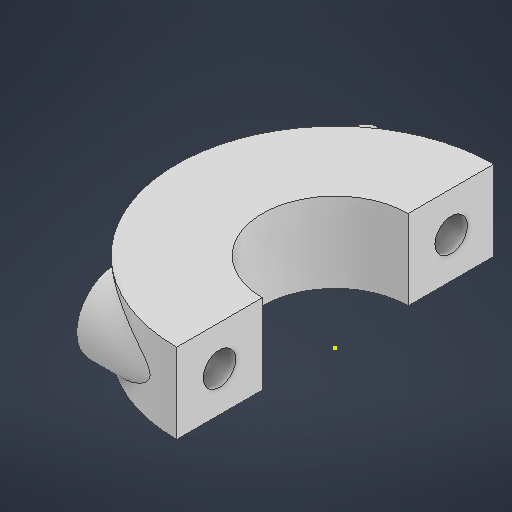
# Autodesk Inventor part: clamp_bolt
Saved by Autodesk Inventor 2026.2 (Build 302298000, 298)
## iProperties
Created: 2026-01-11
Part Number: clamp_bolt
Material: Generic
Document SubType Name: Modeling
Designer: User
Density: 1 g/cm^3
Appearance: Default
Author: User
Autodesk Inventor part; units mm, degrees
ref_plane "YZ Plane" through (0, 0, 0) normal (1, 0, 0) x (0, 1, 0)
ref_plane "XZ Plane" through (0, 0, 0) normal (0, 1, 0) x (-1, 0, 0)
ref_plane "XY Plane" through (0, 0, 0) normal (0, 0, 1) x (1, 0, 0)
sketch "Sketch1" plane through (0, 0, 0) normal (0, 1, 0) x (-1, 0, 0)
  point P0 (0, 0)
sketch "Sketch2" plane through (0, 0, 0) normal (0, 1, 0) x (-1, 0, 0)
  arc A0 (0, -12.775) -> (0, 12.775) centre (0, 0) ccw
  arc A1 (0, -27.775) -> (0, 27.775) centre (0, 0) ccw
  line L0 (0, 27.775) -> (0, -27.775)
  dimension "d0" = 25.55
  dimension "d1" = 15
  constraints: 4 point on circle, 2 centre point, 2 end point, 2 point on line, 1 coincident, 1 vertical
  measures "d0" diameter of A0
  measures "d1" radial gap between concentric circles of A0 A1
extrude "Extrusion1" add sketch "Sketch2" along normal blind 14 contours A0 L0 A1
sketch "Sketch4" plane through (0, 0, 27.775) normal (1, 0, 0) x (0, 0, -1)
  line L0 (4.7364, 11.7377) -> (10.2211, 11.7622)
  line L1 (10.2211, 11.7622) -> (12.9848, 7.0245)
  line L2 (12.9848, 7.0245) -> (10.2636, 2.2623)
  line L3 (10.2636, 2.2623) -> (4.7789, 2.2378)
  line L4 (4.7789, 2.2378) -> (2.0152, 6.9755)
  line L5 (2.0152, 6.9755) -> (4.7364, 11.7377)
  line L6 (0, 14) -> (15, 14) projected
  line L7 (0, 0) -> (0, 14) projected
  line L8 (15, 14) -> (40.55, 14) projected
  line L9 (27.775, 14) -> (27.775, 0)
  line L10 (50.8136, 11.7377) -> (45.3289, 11.7622)
  line L11 (45.3289, 11.7622) -> (42.5652, 7.0245)
  line L12 (42.5652, 7.0245) -> (45.2864, 2.2623)
  line L13 (45.2864, 2.2623) -> (50.7711, 2.2378)
  line L14 (50.7711, 2.2378) -> (53.5348, 6.9755)
  line L15 (53.5348, 6.9755) -> (50.8136, 11.7377)
  line L16 (55.55, 14) -> (40.55, 14)
  line L17 (55.55, 0) -> (55.55, 14)
  line L18 (40.55, 14) -> (15, 14)
  point P0 (7.5, 7)
  point P1 (7.4787, 11.75)
  point P2 (7.5, 14)
  point P3 (0, 7)
  point P4 (48.05, 7)
  point P5 (48.0713, 11.75)
  point P6 (48.05, 14)
  point P7 (55.55, 7)
  dimension "d5" = 9.5
  dimension "d6" = 0
  dimension "d7" = 0
  constraints: 32 end point, 14 symmetric about line, 4 midpoint, 1 vertical, 13 other
  measures "d5" distance from line of L3 point (7.479, 11.75)
  measures "d6" horizontal distance of point (7.5, 14) point (7.5, 7)
  measures "d7" vertical distance of point (0, 7) point (7.5, 7)
extrude "Extrusion2" cut sketch "Sketch4" against normal through all
sketch "Sketch5" plane through (0, 0, 27.775) normal (1, 0, 0) x (0, 0, -1)
  line L0 (4.7364, 11.7377) -> (10.2211, 11.7622) projected
  circle A0 centre (7.4787, 6.9999) radius 2.85
  line L1 (0.8522, 11.9261) -> (14.3606, 11.9261)
  line L2 (14.3606, 11.9261) -> (14.3606, 2.2036)
  line L3 (14.3606, 2.2036) -> (0.8522, 2.2036)
  line L4 (0.8522, 2.2036) -> (0.8522, 11.9261)
  line L5 (10.2636, 2.2623) -> (4.7789, 2.2378) projected
  line L6 (55.55, 14) -> (0, 14) projected
  line L7 (27.775, 14) -> (27.775, 0)
  line L8 (55.55, 0) -> (0, 0) projected
  line L9 (50.8136, 11.7377) -> (45.3289, 11.7622)
  circle A1 centre (48.0713, 6.9999) radius 2.85
  line L10 (54.6978, 11.9261) -> (41.1894, 11.9261)
  line L11 (41.1894, 11.9261) -> (41.1894, 2.2036)
  line L12 (41.1894, 2.2036) -> (54.6978, 2.2036)
  line L13 (54.6978, 2.2036) -> (54.6978, 11.9261)
  line L14 (45.2864, 2.2623) -> (50.7711, 2.2378)
  point P0 (7.4787, 11.75)
  point P1 (7.4787, 11.75)
  point P2 (48.0713, 11.75)
  point P3 (48.0713, 11.75)
  dimension "d12" = 5.7
  dimension "d13" = 0
  dimension "d14" = 4.75
  constraints: 22 end point, 11 symmetric about line, 4 midpoint, 2 centre point, 2 parallel, 1 horizontal, 1 perpendicular, 1 other
  measures "d12" diameter of A0
  measures "d13" horizontal distance of point (7.479, 11.75) A0.centre
  measures "d14" distance from line of L5 A0.centre
extrude "Extrusion3" add sketch "Sketch5" against normal blind 6
sketch "Sketch6" plane through (-6, 0, 27.775) normal (-1, 0, 0) x (0, 0, 1)
  line L0 (-27.775, 0) -> (-27.775, 14)
  line L1 (-40.55, 14) -> (-15, 14) projected
  line L2 (-10.2636, 2.2623) -> (-4.7789, 2.2378) projected
  line L3 (-10.2636, 2.2623) -> (-4.7789, 2.2378)
  line L4 (-4.7789, 2.2378) -> (-2.0152, 6.9755) projected
  line L5 (-4.7789, 2.2378) -> (-2.0152, 6.9755)
  line L6 (-2.0152, 6.9755) -> (-4.7364, 11.7377) projected
  line L7 (-2.0152, 6.9755) -> (-4.7364, 11.7377)
  line L8 (-4.7364, 11.7377) -> (-10.2636, 11.7624)
  line L9 (-10.2636, 11.7624) -> (-13.0059, 7.0615)
  line L10 (-13.0059, 7.0615) -> (-10.2636, 2.2623)
  circle A0 centre (-7.4787, 6.9999) radius 2.85 projected
  circle A1 centre (-7.4787, 6.9999) radius 7
  line L11 (-45.2864, 2.2623) -> (-50.7711, 2.2378)
  line L12 (-45.2864, 2.2623) -> (-50.7711, 2.2378)
  line L13 (-50.7711, 2.2378) -> (-53.5348, 6.9755)
  line L14 (-50.7711, 2.2378) -> (-53.5348, 6.9755)
  line L15 (-53.5348, 6.9755) -> (-50.8136, 11.7377)
  line L16 (-53.5348, 6.9755) -> (-50.8136, 11.7377)
  line L17 (-50.8136, 11.7377) -> (-45.2864, 11.7624)
  line L18 (-45.2864, 11.7624) -> (-42.5441, 7.0615)
  line L19 (-42.5441, 7.0615) -> (-45.2864, 2.2623)
  circle A2 centre (-48.0713, 6.9999) radius 2.85
  circle A3 centre (-48.0713, 6.9999) radius 7
  dimension "d17" = 14
  constraints: 32 end point, 8 symmetric about line, 3 centre point, 3 collinear, 3 parallel, 2 coincident, 1 midpoint, 2 other
  measures "d17" diameter of A1
extrude "Extrusion4" add sketch "Sketch6" along normal blind 12 and the other way blind 6 contours A1 | A3
body "Solid1"
